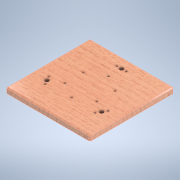
# Autodesk Inventor part: De_Go
Saved by Autodesk Inventor 2022 (Build 260153000, 153)
## iProperties
Created: 2022-11-10
Part Number: De_Go
Material: Wood (Oak)
Document SubType Name: Modeling
Designer: nguye
Density: 0.76 g/cm^3
Appearance: White Oak - Natural Medium Gloss
Author: nguye
Autodesk Inventor part; units mm, degrees
ref_plane "YZ Plane" through (0, 0, 0) normal (1, 0, 0) x (0, 1, 0)
ref_plane "XZ Plane" through (0, 0, 0) normal (0, 1, 0) x (-1, 0, 0)
ref_plane "XY Plane" through (0, 0, 0) normal (0, 0, 1) x (1, 0, 0)
sketch "Sketch1" plane through (0, 0, 0) normal (0, 1, 0) x (-1, 0, 0)
  point P0 (0, 0)
sketch "Sketch2" plane through (0, 0, 0) normal (0, 1, 0) x (-1, 0, 0)
  line L0 (80, -80) -> (-80, -80)
  line L1 (-80, -80) -> (-80, 80)
  line L2 (-80, 80) -> (80, 80)
  line L3 (80, 80) -> (80, -80)
  line L4 (80, -80) -> (-80, 80) construction
  line L5 (-80, -80) -> (80, 80) construction
  point P0 (0, 0)
  dimension "d0" = 160
  dimension "d1" = 160
  constraints: 12 end point, 2 midpoint, 2 parallel, 1 horizontal, 1 perpendicular
  measures "d0" distance of L1.end L2.end
  measures "d1" distance of L0.end L1.end
extrude "Extrusion1" add sketch "Sketch2" along normal blind 10
chamfer "Chamfer1" distance 2 angle 45 8 edges at (80, 10, 0) (0, 10, 80) (80, 5, 80) (80, 5, -80) (-80, 10, 0) (-80, 5, 80) (-80, 5, -80) (0, 10, -80)
sketch "Sketch3" plane through (0, 10, 0) normal (0, 1, 0) x (1, 0, 0)
  point P0 (0, 0)
  point P1 (0, 60)
  point P2 (-51.9615, -30)
  point P3 (51.9615, -30)
  dimension "d8" = 60
  dimension "d11" = 360
  constraints: 1 vertical alignment, 4 other
  measures "d8" distance of point (0, 0) point (0, 60)
hole "Hole1" at (0, 10, -60) at (-51.9615, 10, 30) at (51.9615, 10, 30) direction (0, -1, 0) diameter 8 end through all
sketch "Sketch4" plane through (0, 10, 0) normal (0, 1, 0) x (1, 0, 0)
  circle A0 centre (0, 60) radius 4 projected
  point P0 (0, 0)
  point P1 (-9, 60)
  point P2 (9, 60)
  dimension "d20" = 18
  dimension "d21" = 9
  constraints: 2 horizontal alignment
  measures "d20" distance of point (9, 60) point (-9, 60)
  measures "d21" distance of A0.centre point (9, 60)
hole "Hole2" at (-9, 10, -60) at (9, 10, -60) direction (0, -1, 0) diameter 4 end through all
pattern_circular "Circular Pattern1" count 3 over 360 about axis through (0, -10, 0) along (0, 1, 0) of "Hole2"
sketch "Sketch5" plane through (0, 10, 0) normal (0, 1, 0) x (1, 0, 0)
  point P0 (0, 0)
  point P1 (0, 35)
  dimension "d32" = 35
  constraints: 1 vertical alignment
  measures "d32" distance of point (0, 0) point (0, 35)
hole "Hole3" at (0, 10, -35) direction (0, -1, 0) diameter 4 end through all
pattern_circular "Circular Pattern2" count 6 over 360 about axis through (0, -10, 0) along (0, 1, 0) of "Hole3"
body "Solid1"
